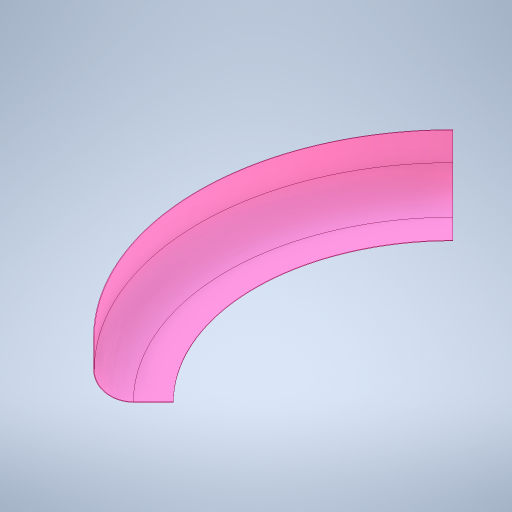
# Autodesk Inventor part: baase
Saved by Autodesk Inventor 2023.2 (Build 272271000, 271)
## iProperties
Created: 2023-01-07
Part Number: baase
Material: Stainless Steel
Document SubType Name: Modeling
Designer: omrfrkmll
Density: 8 g/cm^3
Appearance: Pink
Author: omrfrkmll
Autodesk Inventor part; units mm, degrees
ref_plane "YZ Plane" through (0, 0, 0) normal (1, 0, 0) x (0, 1, 0)
ref_plane "XZ Plane" through (0, 0, 0) normal (0, 1, 0) x (-1, 0, 0)
ref_plane "XY Plane" through (0, 0, 0) normal (0, 0, 1) x (1, 0, 0)
sketch "Sketch1" plane through (0, 0, 0) normal (0, 1, 0) x (-1, 0, 0)
  line L0 (234.273325, 0) -> (-398.047733, 0)
  line L1 (0, 269.522777) -> (0, -364.967462)
  line L2 (250, 500) -> (-250, 500)
  line L3 (-250, 500) -> (-250, -500)
  line L4 (-250, -500) -> (250, -500)
  line L5 (250, -500) -> (250, 500)
  point P0 (0, 0)
  dimension "d0" = 1000
  dimension "d1" = 500
  constraints: 12 end point, 2 horizontal, 2 parallel, 2 point on line, 1 perpendicular, 1 vertical, 2 other
  measures "d0" distance between parallel lines of L4 L2
  measures "d1" distance between parallel lines of L3 L5
sketch "Sketch1 outline for Extrusion1" plane through (0, 0, 0) normal (0, 1, 0) x (-1, 0, 0)
  line L0 (250, -500) -> (250, 500)
  line L1 (-250, -500) -> (250, -500)
  line L2 (-250, 500) -> (-250, -500)
  line L3 (250, 500) -> (-250, 500)
extrude "Extrusion1" add sketch "Sketch1 outline for Extrusion1" along normal blind 10
fillet "Fillet1" radius 2 1 edges at (250, 10, 0)
sketch "Sketch4" plane through (0, 0, 0) normal (0, 0, 1) x (1, 0, 0)
  line L0 (-250, 0) -> (250, 0)
  arc A0 (-750, 500) -> (-250, 0) centre (-250, 500) ccw
  line L1 (-750, 500) -> (-750, 1000)
  line L2 (-250, 0) -> (-250, 10)
  line L3 (-787.939288, 1000) -> (-661.662469, 1000)
  line L4 (-740, 500) -> (-740, 1000)
  arc A1 (-740, 500) -> (-250, 10) centre (-250, 500) ccw
  line L5 (-250, 0) -> (-250, 10)
  line L6 (3750, 901.000805) -> (3750, -131.113672)
  line L7 (-250, 10) -> (250, 10)
  line L8 (-250, 10) -> (248, 10)
  line L9 (250, 10) -> (250, 0)
  line L10 (-250, 0) -> (250, 0)
  point P0 (0, 0)
  dimension "d17" = 500
  dimension "d18" = 10
  dimension "d19" = 1000
  dimension "d20" = 4000
  constraints: 16 end point, 4 point on circle, 3 tangent, 2 centre point, 2 perpendicular, 2 point on line, 2 vertical, 1 coincident, 1 collinear, 1 horizontal, 1 parallel
  measures "d17" distance between parallel lines of L2 L1
  measures "d18" distance between parallel lines of L1 L4
  measures "d19" distance between parallel lines of L0 L3
  measures "d20" distance from line of A0.centre L6
sketch "Sketch4 outline for Revolution1" plane through (0, 0, 0) normal (0, 0, 1) x (1, 0, 0)
  arc A0 (-750, 500) -> (-250, 0) centre (-250, 500) ccw
  line L0 (-250, 0) -> (250, 0)
  line L1 (250, 0) -> (250, 10)
  line L2 (250, 10) -> (-250, 10)
  arc A1 (-250, 10) -> (-740, 500) centre (-250, 500) cw
  line L3 (-740, 500) -> (-740, 1000)
  line L4 (-740, 1000) -> (-750, 1000)
  line L5 (-750, 1000) -> (-750, 500)
revolve "Revolution1" add sketch "Sketch4 outline for Revolution1" angle 90 mid plane about axis through (3750, 901.000805, 0) along (0, -1, 0)
body "Solid1"
